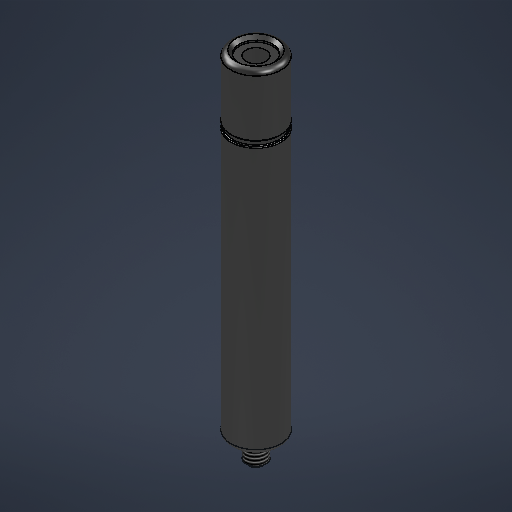
# Autodesk Inventor part: Cylinder
Saved by Autodesk Inventor 2026 (Build 300175050, 175E)
## iProperties
Created: 2025-07-03
Part Number: Cylinder
Material: Stainless Steel
Document SubType Name: Modeling
Designer: Joshua Eah
Density: 8 g/cm^3
Appearance: Glossy - Black
Author: Joshua Eah
Autodesk Inventor part; units mm, degrees
ref_plane "YZ Plane" through (0, 0, 0) normal (1, 0, 0) x (0, 1, 0)
ref_plane "XZ Plane" through (0, 0, 0) normal (0, 1, 0) x (-1, 0, 0)
sketch "Sketch1" plane through (0, 0, 0) normal (0, 1, 0) x (-1, 0, 0)
  circle A0 centre (0, 0) radius 7.5
  circle A1 centre (0, 0) radius 3
  dimension "d0" = 15
  dimension "d3" = 6
  constraints: 2 centre point, 2 coincident
  measures "d0" diameter of A0
  measures "d3" diameter of A1
extrude "Extrusion1" add sketch "Sketch1" along normal blind 100 contours A0 | A1
extrude "Extrusion2" add sketch "Sketch1" against normal blind 7 contours A1
sketch "Sketch2" plane through (0, 100, 0) normal (0, 1, 0) x (1, 0, 0)
  circle A0 centre (0, 0) radius 3 projected
  circle A1 centre (0, 0) radius 3
  circle A2 centre (0, 0) radius 5
  dimension "d6" = 6
  dimension "d20" = 10
  constraints: 2 centre point, 2 coincident
  measures "d6" diameter of A1
  measures "d20" diameter of A2
hole "Hole1" at (0, 100, 0) direction (0, -1, 0) diameter 6 depth 70
ref_plane "Work Plane1" through (0, 81.5, 0) normal (0, 1, 0) x (1, 0, 0)
sketch "Sketch3" plane through (0, 81.5, 0) normal (0, 1, 0) x (1, 0, 0)
  circle A0 centre (0, 0) radius 3 projected
  circle A1 centre (0, 0) radius 7
  circle A2 centre (0, 0) radius 7.5
  dimension "d27" = 14
  constraints: 2 centre point, 2 coincident
  measures "d27" diameter of A1
extrude "Extrusion4" cut sketch "Sketch3" against normal blind 1.5 contours A2
fillet "Fillet2" radius 0.25 4 edges at (-7, 81.5, 0) (-7, 80, 0) (7.5, 81.5, 0) (7.5, 80, 0)
thread "Thread1" size "M6x1" class "6g" standard "ANSI Metric M Profile" full length
fillet "Fillet1" radius 1.5 2 edges at (7.5, 0, 0) (7.5, 100, 0)
chamfer "Chamfer1" distance 1 angle 45 1 edges at (3, -7, 0)
extrude "Extrusion3" cut sketch "Sketch2" against normal blind 1.5
chamfer "Chamfer2" distance 1 angle 45 1 edges at (-5, 100, 0)
body "Solid1"
